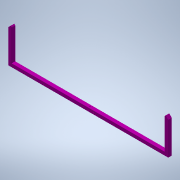
# Autodesk Inventor part: BASE_FUNDO_SUPORTE_LAMINA
Saved by Autodesk Inventor 2021 (Build 250183000, 183)
## iProperties
Created: 2016-02-21
Part Number: BASE_FUNDO_SUPORTE_LAMINA
Material: Genérico
Document SubType Name: Modeling
Designer: Everton
Density: 1 g/cm^3
Appearance: Padrão
Author: Everton
Autodesk Inventor part; units mm, degrees
ref_plane "YZ Plane" through (0, 0, 0) normal (1, 0, 0) x (0, 1, 0)
ref_plane "XZ Plane" through (0, 0, 0) normal (0, 1, 0) x (-1, 0, 0)
ref_plane "XY Plane" through (0, 0, 0) normal (0, 0, 1) x (1, 0, 0)
sketch "Sketch1" plane through (0, 0, 0) normal (0, 1, 0) x (-1, 0, 0)
  line L0 (3880.5632, 208.6837) -> (3853.3913, 235.9005)
  arc A0 (3880.5632, 208.6837) -> (3881.9735, 208.0967) centre (3881.9785, 210.0967) ccw
  line L1 (2078.8655, 206.2751) -> (2106.1695, 233.5659)
  arc A1 (2077.4795, 205.6899) -> (2078.8655, 206.2751) centre (2077.4516, 207.6897) ccw
  arc A2 (3883.0351, 262.7329) -> (3883.0378, 262.7357) centre (2978.5428, 1160.9837) ccw
  arc A3 (3881.9735, 261.6652) -> (3881.9774, 261.6692) centre (2978.5428, 1160.9837) ccw
  line L2 (2979.7274, -125.1538) -> (3881.9735, -125.1538)
  line L3 (3879.7274, -165.1538) -> (2079.7274, -165.1538)
  line L4 (2079.7274, -125.1538) -> (2979.7274, -125.1538)
  line L5 (3879.7274, -165.1538) -> (3881.9735, -165.1538)
  line L6 (2079.7274, -165.1538) -> (2077.4795, -165.1538)
  line L7 (2117.4795, -125.1538) -> (2077.4795, -125.1538)
  line L8 (2089.1735, -125.1538) -> (3870.2812, -125.1538)
  line L9 (2077.4795, 205.6899) -> (2077.4795, -165.1538)
  line L10 (2117.4795, 223.0557) -> (2117.4795, -125.1538)
  line L11 (3881.9735, 208.0967) -> (3881.9735, -165.1538)
  line L12 (3841.9735, 225.2347) -> (3841.9735, -125.1538)
  line L13 (3841.9735, -125.1538) -> (3881.9735, -125.1538)
  arc A4 (3841.9735, 225.2347) -> (3853.3913, 235.9005) centre (2978.5428, 1160.9837) ccw
  line L14 (2117.4795, 223.0557) -> (2106.1695, 233.5659)
  line L15 (3039.7274, -165.1538) -> (3039.7274, -145.1538)
  circle A5 centre (3039.7274, -145.1538) radius 5
  circle A6 centre (2919.7274, -145.1538) radius 5
  point P0 (0, 0)
  point P1 (2077.4509, 204.8613)
  point P2 (2106.1378, 233.5957)
  point P3 (2712.3694, -125.1538)
  dimension "d20" = 40
  dimension "d21" = 40
  constraints: 32 end point, 10 point on circle, 7 centre point, 6 point on line, 1 coincident, 1 horizontal, 1 vertical
  measures "d20" distance between parallel lines of L9 L10
  measures "d21" distance between parallel lines of L11 L12
extrude "Extrusion1" add sketch "Sketch1" along normal blind 40 contours A0 L11 L2 L12 A4 L0 | L11 L5 L3 L6 L9 L7 L4 L2 | L4 L7 L9 A1 L1 L14 L10 | A5 | A6
fillet "Fillet1" radius 2 10 edges at (-3841.9735, 40, 50.0404) (-2979.7265, 40, -125.1538) (-3881.9735, 40, -145.1538) (-3881.9735, 40, 41.4714) (-2978.6034, 40, -165.1538) (-2077.4795, 40, 40.268) (-2077.4795, 40, -145.1538) (-2117.4795, 40, 48.9509) (-3841.9735, 0, 50.0404) (-2979.7265, 0, -125.1538)
fillet "Fillet2" radius 2 9 edges at (-2077.4795, 0, 40.268) (-2077.4795, 0, -145.1538) (-2978.6034, 0, -165.1538) (-2078.0653, 39.4142, -164.568) (-2077.4795, 19, -165.1538) (-3881.3877, 39.4142, -164.568) (-3881.9735, 19, -165.1538) (-3881.9735, 0, 41.4714) (-3881.9735, 0, -145.1538)
sketch "Sketch2" plane through (-2079.4795, 2, -165.1538) normal (0, 0, -1) x (-1, 0, 0)
  line L0 (0, 0) -> (0, 36) projected
  line L1 (0, 18) -> (1800.494, 18)
  line L2 (1800.494, 36) -> (1800.494, 0) projected
  circle A0 centre (900.247, 18) radius 5
  point P0 (-2079.4795, -2)
  dimension "d27" = 10
  constraints: 3 midpoint, 2 end point, 1 centre point
  measures "d27" diameter of A0
extrude "Extrusion2" cut sketch "Sketch2" against normal blind 50
extrude "Extrusion3" cut sketch "Sketch1" along normal blind 60 contours A5 | A6
body "Solid1"
